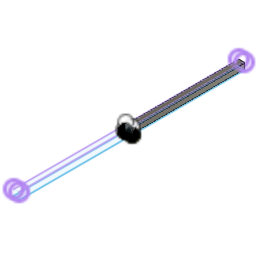
Picture Stand Poles v3 (Autodesk Fusion 360 design; units mm, degrees)
Autodesk Fusion 360 part; units mm, degrees
sketch "Sketch1" plane through (0, 0, 0) normal (0, 0, 1) x (1, 0, 0)
  line L0 (-77.3846, -285.6532) -> (-87.3846, -285.6532)
  line L1 (-77.3846, 64.3468) -> (-77.3846, -285.6532)
  line L2 (-87.3846, -285.6532) -> (-87.3846, 64.3468)
  line L3 (-87.3846, 64.3468) -> (-77.3846, 64.3468)
  dimension "d11" = 10
  dimension "d12" = 350
  constraint horizontal L3
  constraint vertical L1
  constraint horizontal L0
  constraint vertical L2
  measures "d11" distance of L1.start L2.end
  measures "d12" distance of L2.end L0.end
extrude "Extrude3" add sketch "Sketch1" along normal blind 10
fillet "Fillet3" radius 1 2 edges at (-77.3846, -110.6532, 10) (-87.3846, -110.6532, 10)
fillet "Fillet4" radius 1 2 edges at (-77.3846, -110.6532, 0) (-87.3846, -110.6532, 0)
sketch "Sketch2" plane through (0, -285.6532, 0) normal (0, -1, 0) x (1, 0, 0)
  arc A0 (-87.3846, 1) -> (-86.3846, 0) centre (-86.3846, 1) ccw
  line L0 (-86.3846, 0) -> (-78.3846, 0)
  arc A1 (-78.3846, 0) -> (-77.3846, 1) centre (-78.3846, 1) ccw
  line L1 (-77.3846, 1) -> (-77.3846, 9)
  arc A2 (-77.3846, 9) -> (-78.3846, 10) centre (-78.3846, 9) ccw
  line L2 (-78.3846, 10) -> (-86.3846, 10)
  arc A3 (-86.3846, 10) -> (-87.3846, 9) centre (-86.3846, 9) ccw
  line L3 (-87.3846, 9) -> (-87.3846, 1)
  line L4 (-77.3846, 0, -175) -> (-77.3846, 7, -175)
  line L5 (-78.3846, 10, -350) -> (-78.3846, 10, 0)
  line L6 (-86.3846, 10, 0) -> (-86.3846, 10, -350)
  line L7 (-78.3846, 10, -175) -> (-86.3846, 10, -175)
  line L8 (-77.3846, 7, -175) -> (-77.3846, 11, -175)
  line L9 (-78.3846, 10, -175) -> (-77.3846, 10, -175)
  line L10 (-87.3846, 0, -175) -> (-90.5, 0, -175)
  line L11 (-87.3846, 0, -175) -> (-87.3846, 12, -175)
  line L12 (-86.3846, 10, -175) -> (-87.3846, 10, -175)
  line L13 (-87.3846, 0, -175) -> (-77.3846, 0, -175)
  point P0 (-77.3846, 0)
  point P1 (-87.3846, 0)
extrude "Extrude4" cut sketch "Sketch2" against normal blind 175
